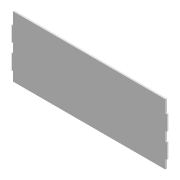
# Autodesk Inventor part: Piso
Saved by Autodesk Inventor 2022 (Build 260153000, 153)
## iProperties
Created: 2022-06-06
Part Number: Piso
Material: Generic
Document SubType Name: Modeling
Designer: ADMIN
Density: 1 g/cm^3
Appearance: Default
Author: ADMIN
Autodesk Inventor part; units mm, degrees
ref_plane "YZ Plane" through (0, 0, 0) normal (1, 0, 0) x (0, 1, 0)
ref_plane "XZ Plane" through (0, 0, 0) normal (0, 1, 0) x (-1, 0, 0)
ref_plane "XY Plane" through (0, 0, 0) normal (0, 0, 1) x (1, 0, 0)
sketch "Sketch1" plane through (0, 0, 0) normal (0, 0, 1) x (1, 0, 0)
  line L0 (505, 160) -> (505, 110) projected
  line L1 (505, 160) -> (500, 160) projected
  line L2 (500, 110) -> (500, 160) projected
  line L3 (505, 110) -> (500, 110) projected
  line L4 (505, 80) -> (505, 30) projected
  line L5 (505, 80) -> (500, 80) projected
  line L6 (500, 30) -> (500, 80) projected
  line L7 (505, 30) -> (500, 30) projected
  line L8 (0, 160) -> (0, 110) projected
  line L9 (0, 160) -> (-5, 160) projected
  line L10 (-5, 110) -> (-5, 160) projected
  line L11 (0, 110) -> (-5, 110) projected
  line L12 (0, 80) -> (0, 30) projected
  line L13 (0, 80) -> (-5, 80) projected
  line L14 (-5, 30) -> (-5, 80) projected
  line L15 (0, 30) -> (-5, 30) projected
  line L16 (-5, 160) -> (0, 160) projected
  line L17 (0, 160) -> (0, 350) projected
  line L18 (0, 350) -> (-5, 350) projected
  line L19 (-5, 160) -> (-5, 350) projected
  line L20 (0, 200) -> (500, 200) projected
  line L21 (500, 200) -> (500, 205) projected
  line L22 (0, 205) -> (500, 205) projected
  line L23 (0, 200) -> (0, 205) projected
  line L24 (500, 160) -> (505, 160) projected
  line L25 (505, 160) -> (505, 350) projected
  line L26 (505, 350) -> (500, 350) projected
  line L27 (500, 160) -> (500, 350) projected
  line L28 (505, 0) -> (500, 0) projected
  line L29 (500, 0) -> (500, -5) projected
  line L30 (505, -5) -> (500, -5) projected
  line L31 (505, 0) -> (505, -5) projected
  line L32 (0, 200) -> (500, 200)
  line L33 (500, 200) -> (500, 0)
  line L34 (500, 0) -> (0, 0)
  line L35 (0, 0) -> (0, 200)
  line L36 (500, 195) -> (0, 195)
  line L37 (0, 5) -> (500, 5)
  point P0 (0, 0)
  point P1 (0, 195)
  dimension "d2" = 5
  dimension "d3" = 5
  constraints: 12 end point, 4 point on line, 3 perpendicular, 2 parallel, 1 horizontal
  measures "d2" distance between parallel lines of L34 L37
  measures "d3" distance between parallel lines of L36 L32
extrude "Extrusion1" add sketch "Sketch1" along normal blind 5 contours L0 L3 L2 L1 | L2 L33 L6 L37 L35 L12 L8 L17 L36 L27 | L5 L4 L7 L6 | L8 L11 L10 L9 | L12 L15 L14 L13
body "Solid1"
